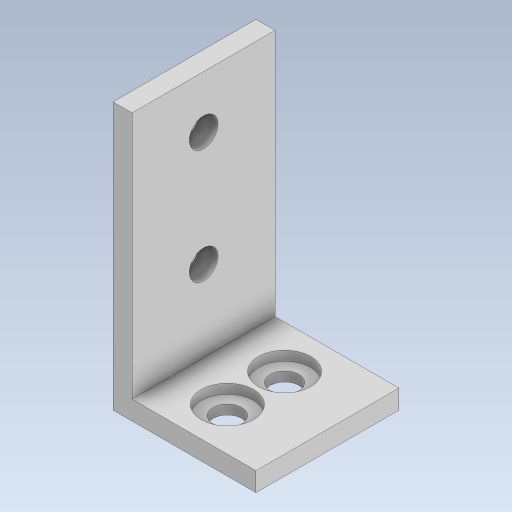
# Autodesk Inventor part: Konektor Lifter 2
Saved by Autodesk Inventor 2023.5 (Build 275446000, 446)
## iProperties
Created: 2025-09-16
Part Number: Konektor Lifter 2
Material: Generic
Document SubType Name: Modeling
Designer: Guntur
Density: 1 g/cm^3
Appearance: Default
Author: Guntur
## iProperties of the stored document Konektor Lifter 2_3DPrint.ipt
Created: 2025-09-20
Part Number: Konektor Lifter 2_3DPrint
Material: Generic
Document SubType Name: Modeling
Designer: Guntur
Density: 1 g/cm^3
Appearance: Default
Author: Guntur
Autodesk Inventor part; units mm, degrees
ref_plane "YZ Plane" through (0, 0, 0) normal (1, 0, 0) x (0, 1, 0)
ref_plane "XZ Plane" through (0, 0, 0) normal (0, 1, 0) x (-1, 0, 0)
ref_plane "XY Plane" through (0, 0, 0) normal (0, 0, 1) x (1, 0, 0)
sketch "Sketch1" plane through (0, 0, 0) normal (0, 1, 0) x (-1, 0, 0)
  line L0 (7.5, 7.5) -> (-7.5, 7.5)
  line L1 (-7.5, 7.5) -> (-7.5, -7.5)
  line L2 (-7.5, -7.5) -> (7.5, -7.5)
  line L3 (7.5, -7.5) -> (7.5, 7.5)
  line L4 (7.5, 7.5) -> (-7.5, -7.5) construction
  line L5 (-7.5, 7.5) -> (7.5, -7.5) construction
  line L6 (7.5, 7.5) -> (5.5, 7.5)
  line L7 (5.5, 7.5) -> (5.5, -7.5)
  line L8 (5.5, -7.5) -> (7.5, -7.5)
  line L9 (7.5, -7.5) -> (7.5, 7.5)
  circle A0 centre (0, 3) radius 1.5
  circle A1 centre (0, 3) radius 2.75
  line L10 (7.5, 0) -> (-7.5, 0) construction
  line L11 (0, 7.5) -> (0, -7.5) construction
  circle A2 centre (0, -3) radius 1.5
  circle A3 centre (0, -3) radius 2.75
  point P0 (0, 0)
  dimension "d0" = 15
  dimension "d1" = 15
  dimension "d2" = 2
  dimension "d3" = 3
  dimension "d4" = 5.5
  dimension "d5" = 4.5
  constraints: 24 end point, 6 midpoint, 4 centre point, 4 parallel, 2 coincident, 2 horizontal, 2 perpendicular, 2 symmetric about line, 1 point on line, 2 other
  measures "d0" distance of L2.end L1.end
  measures "d1" distance of L1.end L0.end
  measures "d2" distance of L8.end L7.end
  measures "d3" diameter of A0
  measures "d4" diameter of A1
  measures "d5" distance from line of L0 A0.centre
extrude "Extrusion1" add sketch "Sketch1" along normal blind 2 contours L7 L2 L1 L0
extrude "Extrusion2" add sketch "Sketch1" along normal blind 1 contours A1 | A3
extrude "Extrusion3" add sketch "Sketch1" along normal blind 28 contours L3 L2 L7 L0
sketch "Sketch2" plane through (-5.5, 2, -7.5) normal (1, 0, 0) x (0, 0, -1)
  circle A0 centre (-7.5, 8.5) radius 1.5
  line L0 (-15, 0) -> (0, 0) projected
  circle A1 centre (-7.5, 20.5) radius 1.5
  point P0 (-7.5, -2)
  dimension "d12" = 3
  dimension "d13" = 8.5
  dimension "d14" = 3
  dimension "d15" = 20.5
  constraints: 2 centre point
  measures "d12" diameter of A0
  measures "d13" distance from line of L0 A0.centre
  measures "d14" diameter of A1
  measures "d15" distance from line of L0 A1.centre
extrude "Extrusion4" cut sketch "Sketch2" against normal blind 2
body "Solid1"
